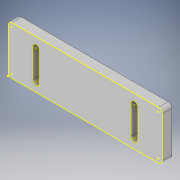
# Autodesk Inventor part: BasePatasVTOL2
Saved by Autodesk Inventor 2019 (Build 230136000, 136)
## iProperties
Created: 2019-04-08
Part Number: BasePatasVTOL2
Material: Generic
Document SubType Name: Modeling
Designer: Kenny
Density: 1 g/cm^3
Appearance: Default
Author: Kenny
Autodesk Inventor part; units mm, degrees
ref_plane "YZ Plane" through (0, 0, 0) normal (1, 0, 0) x (0, 1, 0)
ref_plane "XZ Plane" through (0, 0, 0) normal (0, 1, 0) x (-1, 0, 0)
ref_plane "XY Plane" through (0, 0, 0) normal (0, 0, 1) x (1, 0, 0)
sketch "Sketch1" plane through (0, 0, 0) normal (0, 0, 1) x (1, 0, 0)
  line L0 (0, 0) -> (80, 0)
  line L1 (80, 0) -> (80, 25)
  line L2 (80, 25) -> (0, 25)
  line L3 (0, 25) -> (0, 0)
  point P0 (14.5, 19.7286)
  point P1 (14.5, 4.7286)
  point P2 (65.5, 19.7286)
  point P3 (65.5, 4.7286)
  dimension "d0" = 80
  dimension "d1" = 25
  dimension "d2" = 14.5
  dimension "d3" = 51
  dimension "d4" = 15
  constraints: 8 end point, 2 horizontal alignment, 2 parallel, 2 vertical alignment, 1 horizontal, 1 perpendicular
  measures "d0" distance of L2.end L1.end
  measures "d1" distance of L1.end L0.end
  measures "d2" distance from line of L3 point (14.5, 19.729)
  measures "d3" distance of point (65.5, 19.729) point (14.5, 19.729)
  measures "d4" distance of point (14.5, 4.729) point (14.5, 19.729)
extrude "Extrusion1" add sketch "Sketch1" along normal blind 5
sketch "Sketch2" plane through (0, 0, 0) normal (0, 0, 1) x (1, 0, 0)
  line L0 (0, 0) -> (80, 0)
  line L1 (80, 0) -> (80, 25)
  line L2 (80, 25) -> (0, 25)
  line L3 (0, 25) -> (0, 0)
  point P0 (14.5, 19.7286)
  point P1 (14.5, 4.7286)
  point P2 (65.5, 19.7286)
  point P3 (65.5, 4.7286)
  dimension "d5" = 80
  dimension "d6" = 25
  dimension "d7" = 14.5
  dimension "d8" = 51
  dimension "d9" = 15
  constraints: 8 end point, 2 horizontal alignment, 2 parallel, 2 vertical alignment, 1 horizontal, 1 perpendicular
  measures "d5" distance of L2.end L1.end
  measures "d6" distance of L1.end L0.end
  measures "d7" distance from line of L3 point (14.5, 19.729)
  measures "d8" distance of point (65.5, 19.729) point (14.5, 19.729)
  measures "d9" distance of point (14.5, 4.729) point (14.5, 19.729)
hole "Hole1" at (14.5, 19.7286, 0) at (14.5, 4.7286, 0) at (65.5, 19.7286, 0) at (65.5, 4.7286, 0) direction (0, 0, 1) diameter 3.5 end through all
sketch "Sketch3" plane through (0, 0, 5) normal (0, 0, 1) x (1, 0, 0)
  circle A0 centre (14.5, 19.7286) radius 1.75 projected
  line L0 (16.25, 19.7286) -> (16.25, 4.7286)
  line L1 (12.75, 19.7286) -> (12.75, 4.7286)
  circle A1 centre (14.5, 4.7286) radius 1.75 projected
  circle A2 centre (65.5, 19.7286) radius 1.75 projected
  line L2 (63.75, 19.7286) -> (63.75, 4.7286)
  line L3 (67.25, 19.7286) -> (67.25, 4.7286)
  circle A3 centre (65.5, 4.7286) radius 1.75 projected
  circle A4 centre (65.5, 19.7286) radius 1.75 projected
  circle A5 centre (65.5, 4.7286) radius 1.75 projected
  circle A6 centre (14.5, 19.7286) radius 1.75 projected
  circle A7 centre (14.5, 4.7286) radius 1.75 projected
  point P0 (0, 0)
  constraints: 8 end point, 8 tangent, 6 point on circle, 4 vertical, 1 horizontal alignment, 1 other
extrude "Extrusion2" cut sketch "Sketch3" against normal blind 5 contours L0 A1 L1 A0 | L3 A3 L2 A2
fillet "Fillet1" radius 2 4 edges at (80, 25, 2.5) (80, 0, 2.5) (0, 25, 2.5) (0, 0, 2.5)
sketch "Sketch4" plane through (0, 0, 5) normal (0, 0, 1) x (1, 0, 0)
  line L0 (63.75, 4.7286) -> (63.75, 19.7286) projected
  arc A0 (67.25, 19.7286) -> (63.75, 19.7286) centre (65.5, 19.7286) ccw projected
  line L1 (67.25, 19.7286) -> (67.25, 4.7286) projected
  arc A1 (63.75, 4.7286) -> (67.25, 4.7286) centre (65.5, 4.7286) ccw projected
  line L2 (12.75, 4.7286) -> (12.75, 19.7286) projected
  arc A2 (16.25, 19.7286) -> (12.75, 19.7286) centre (14.5, 19.7286) ccw projected
  line L3 (16.25, 19.7286) -> (16.25, 4.7286) projected
  arc A3 (12.75, 4.7286) -> (16.25, 4.7286) centre (14.5, 4.7286) ccw projected
  arc A4 (0, 2) -> (2, 0) centre (2, 2) ccw projected
  line L4 (2, 0) -> (78, 0) projected
  arc A5 (78, 0) -> (80, 2) centre (78, 2) ccw projected
  line L5 (80, 2) -> (80, 23) projected
  arc A6 (80, 23) -> (78, 25) centre (78, 23) ccw projected
  line L6 (78, 25) -> (2, 25) projected
  arc A7 (2, 25) -> (0, 23) centre (2, 23) ccw projected
  line L7 (0, 23) -> (0, 2) projected
  point P0 (0, 0)
body "Solid1"
